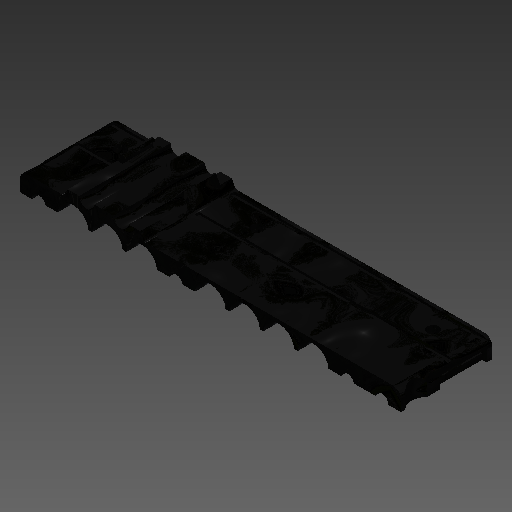
# Autodesk Inventor part: 3d_LM - Pinza 2
Saved by Autodesk Inventor 2018.3 (Build 223284000, 284)
## iProperties
Created: 2026-02-09
Part Number: 3d_LM - Pinza 2
Material: PA12 SLS 3D Print
Document SubType Name: Modeling
Designer: aca6
Density: 0.95 g/cm^3
Appearance: Black
Manufacturer-1: {"Name": "BERNARDO HENAREJOS ORENES (TECNOBRO)", "PartNumber": "3d_LM - Pinza 2", "Link": ""}
Manufacturer-2: {"Name": "MATERIALISE NV", "PartNumber": "3d_LM - Pinza 2", "Link": ""}
Manufacturer-3: {"Name": "", "PartNumber": "", "Link": ""}
Manufacturer-4: {"Name": "", "PartNumber": "", "Link": ""}
Manufacturer-5: {"Name": "", "PartNumber": "", "Link": ""}
Provider-1: {"Name": "", "PartNumber": "", "Link": ""}
Provider-2: {"Name": "", "PartNumber": "", "Link": ""}
Provider-3: {"Name": "", "PartNumber": "", "Link": ""}
Provider-4: {"Name": "", "PartNumber": "", "Link": ""}
Provider-5: {"Name": "", "PartNumber": "", "Link": ""}
Author: aca6
Comments: DIN-ISO-2768-mK
Autodesk Inventor part; units mm, degrees
ref_plane "YZ Plane" through (0, 0, 0) normal (1, 0, 0) x (0, 1, 0)
ref_plane "XZ Plane" through (0, 0, 0) normal (0, 1, 0) x (-1, 0, 0)
ref_plane "XY Plane" through (0, 0, 0) normal (0, 0, 1) x (1, 0, 0)
sketch "Sketch1" plane through (0, 0, 0) normal (0, 0, 1) x (1, 0, 0)
  arc A0 (-21.6, 0) -> (-23.4, 0) centre (-22.5, 0) ccw
  arc A1 (-15.975, 0) -> (-20.025, 0) centre (-18, 0) ccw
  arc A2 (-11.475, 0) -> (-15.525, 0) centre (-13.5, 0) ccw
  arc A3 (-6.975, 0) -> (-11.025, 0) centre (-9, 0) ccw
  arc A4 (-3.6, 0) -> (-5.4, 0) centre (-4.5, 0) ccw
  arc A5 (2.025, 0) -> (-2.025, 0) centre (0, 0) ccw
  arc A6 (6.525, 0) -> (2.475, 0) centre (4.5, 0) ccw
  arc A7 (11.025, 0) -> (6.975, 0) centre (9, 0) ccw
  arc A8 (15.525, 0) -> (11.475, 0) centre (13.5, 0) ccw
  arc A9 (18.875, 0) -> (17.125, 0) centre (18, 0) ccw
  arc A10 (23.375, 0) -> (21.625, 0) centre (22.5, 0) ccw
  line L0 (-25, 0) -> (-25, 1.5)
  line L1 (-25, 0) -> (25, 0)
  line L2 (25, 0) -> (25, 1.5)
  arc A11 (25, 1.5) -> (24, 2.5) centre (24, 1.5) ccw
  arc A12 (-24, 2.5) -> (-25, 1.5) centre (-24, 1.5) ccw
  line L3 (-8.467, 2.5) -> (24, 2.5)
  line L4 (-19.1661, 2.65) -> (-18.6985, 3.46)
  line L5 (-18.6985, 3.46) -> (-9.1945, 3.46)
  line L6 (-9.1945, 3.46) -> (-8.7268, 2.65)
  line L7 (-9.1945, 3.46) -> (-8.2592, 3.46) construction
  arc A13 (-8.7268, 2.65) -> (-8.467, 2.5) centre (-8.467, 2.8) ccw
  line L8 (-19.4259, 2.5) -> (-24, 2.5)
  arc A14 (-19.4259, 2.5) -> (-19.1661, 2.65) centre (-19.4259, 2.8) ccw
  line L9 (0, 0) -> (0, 12.7088) construction
  point P0 (-19.2527, 2.5)
  point P1 (-8.6402, 2.5)
  dimension "d1" = 1.8
  dimension "d2" = 4.5
  dimension "d3" = 4.5
  dimension "d4" = 4.5
  dimension "d5" = 4.5
  dimension "d6" = 4.5
  dimension "d7" = 4.5
  dimension "d8" = 4.5
  dimension "d9" = 4.5
  dimension "d10" = 4.5
  dimension "d11" = 4.5
  dimension "d12" = 4.05
  dimension "d13" = 4.05
  dimension "d14" = 4.05
  dimension "d15" = 1.8
  dimension "d16" = 4.05
  dimension "d17" = 4.05
  dimension "d18" = 4.05
  dimension "d19" = 4.05
  dimension "d20" = 1.75
  dimension "d21" = 1.75
  dimension "d22" = 2.5
  dimension "d23" = 50
  dimension "d24" = 1.5
  dimension "d25" = 1.5
  dimension "d26" = 1
  dimension "d27" = 1
  dimension "d29" = 120
  dimension "d32" = 9.504
  dimension "d33" = 60
  dimension "d67" = 0.96
  dimension "d68" = 0.3
  dimension "d69" = 0.3
  dimension "d70" = 33.467
  dimension "d71" = 5.5741
  constraints: 30 point on circle, 18 end point, 15 centre point, 9 tangent, 6 point on line, 4 vertical, 2 horizontal, 1 equal length, 39 other
  measures "d1" diameter of A0
  measures "d2" distance of A1.centre A0.centre
  measures "d3" distance of A2.centre A1.centre
  measures "d4" distance of A2.centre A3.centre
  measures "d5" distance of A3.centre A4.centre
  measures "d6" distance of A4.centre A5.centre
  measures "d7" distance of A5.centre A6.centre
  measures "d8" distance of A7.centre A6.centre
  measures "d9" distance of A8.centre A7.centre
  measures "d10" distance of A9.centre A8.centre
  measures "d11" distance of A10.centre A9.centre
  measures "d12" diameter of A1
  measures "d13" diameter of A2
  measures "d14" diameter of A3
  measures "d15" diameter of A4
  measures "d16" diameter of A5
  measures "d17" diameter of A6
  measures "d18" diameter of A7
  measures "d19" diameter of A8
  measures "d20" diameter of A9
  measures "d21" diameter of A10
  measures "d22" distance from line of A0.centre L0
  measures "d23" distance of L0.start L2.start
  measures "d24" distance of L0.start L0.end
  measures "d25" distance of L2.start L2.end
  measures "d26" radius of A11
  measures "d27" radius of A12
  measures "d29" angle of L3 L4
  measures "d32" distance of L4.end L5.end
  measures "d33" angle of L6 L7
  measures "d67" distance from line of L3 L5.end
  measures "d68" radius of A13
  measures "d69" radius of A14
  measures "d70" distance from line of L2 L3.start
  measures "d71" distance from line of L0 L8.start
extrude "Extrusion1" add sketch "Sketch1" along normal blind 12 contours A0 L1 L0 A12 L8 A14 L4 L5 L6 A13 L3 A11 L2 A10 A9 A8 A7 A6 A5 A4 A3 A2 A1
sketch "Sketch2" plane through (0, 0, 12) normal (0, 0, 1) x (1, 0, 0)
  line L0 (-9.1945, 3.46) -> (-18.6985, 3.46) projected
  point P0 (0, 0)
  point P1 (-16.1965, 3.46)
  point P2 (-11.6965, 3.46)
  dimension "d39" = 4.5
  dimension "d40" = 2.502
  constraints: 2 point on line
  measures "d39" distance of point (-11.696, 3.46) point (-16.196, 3.46)
  measures "d40" distance of L0.end point (-16.196, 3.46)
hole "Hole1" at (-16.1965, 3.46, 12) at (-11.6965, 3.46, 12) direction (0, 0, -1) diameter 2 end through all
sketch "Sketch3" plane through (24, 2.5, 12) normal (0, 1, 0) x (1, 0, 0)
  line L0 (0.714, 6.4) -> (-32.467, 6.4)
  line L1 (-32.467, 6.4) -> (-32.467, 7)
  line L2 (-32.467, 7) -> (0.714, 7)
  line L3 (0.714, 7) -> (0.714, 6.4)
  line L4 (-32.467, 11) -> (0.714, 11)
  line L5 (0.714, 11) -> (0.714, 11.6)
  line L6 (0.714, 11.6) -> (-32.467, 11.6)
  line L7 (-32.467, 11.6) -> (-32.467, 11)
  line L8 (1, 12) -> (1, 0) projected
  line L9 (0, 12) -> (-32.467, 12) projected
  line L10 (-43.4259, 6.4) -> (-48.29, 6.4)
  line L11 (-48.29, 6.4) -> (-48.29, 7)
  line L12 (-48.29, 7) -> (-43.4259, 7)
  line L13 (-43.4259, 7) -> (-43.4259, 6.4)
  line L14 (-43.4259, 11.6) -> (-48.29, 11.6)
  line L15 (-48.29, 11.6) -> (-48.29, 11)
  line L16 (-48.29, 11) -> (-43.4259, 11)
  line L17 (-43.4259, 11) -> (-43.4259, 11.6)
  line L18 (-49, 12) -> (-49, 0) projected
  point P0 (-24, 12)
  point P1 (-32.5535, 12.5)
  point P2 (-32.467, 12)
  point P3 (-43.4259, 12)
  dimension "d48" = 0.286
  dimension "d49" = 0.286
  dimension "d50" = 0.6
  dimension "d51" = 0.6
  dimension "d57" = 0.4
  dimension "d58" = 4
  dimension "d79" = 0.71
  constraints: 32 end point, 8 parallel, 5 point on line, 4 horizontal, 4 horizontal alignment, 4 perpendicular, 1 other
  measures "d48" distance between parallel lines of L8 L3
  measures "d49" distance between parallel lines of L8 L5
  measures "d50" distance of L2.end L0.start
  measures "d51" distance of L4.end L5.end
  measures "d58" distance between parallel lines of L2 L4
  measures "d79" distance between parallel lines of L18 L11
extrude "Extrusion2" cut sketch "Sketch3" against normal blind 0.3
ref_plane "Work Plane1" through (-2.9282, 3.7996, 12.5) normal (0, 1, 0) x (1, 0, 0)
sketch "Sketch4" plane through (-2.9282, 2.5, 12.5) normal (0, 1, 0) x (1, 0, 0)
  line L0 (27.9282, 12.5495) -> (27.9282, 3.2148)
  line L1 (26.9282, 11.5) -> (-5.5388, 11.5) projected
  line L2 (27.9282, 12.5) -> (27.9282, 0.5) projected
  line L3 (-22.0718, 12.5) -> (-22.0718, 0.5) projected
  point P0 (2.9282, 12.5)
  point P1 (-17.8838, 9.5)
  point P2 (0.1157, 9.5)
  point P3 (23.1782, 9.5)
  dimension "d54" = 4.75
  dimension "d72" = 2
  dimension "d121" = 4.188
  dimension "d122" = 23.0625
  constraints: 2 end point, 2 horizontal alignment, 2 point on line
  measures "d54" distance from line of L0 point (23.178, 9.5)
  measures "d72" distance from line of L1 point (23.178, 9.5)
  measures "d121" distance from line of L3 point (-17.884, 9.5)
  measures "d122" distance of point (0.116, 9.5) point (23.178, 9.5)
hole "Hole2" at (-20.812, 2.5, 3) at (-2.8125, 2.5, 3) at (20.25, 2.5, 3) direction (0, -1, 0) diameter 1.5 end through all both
sketch "Sketch5" plane through (-8.467, 2.5, 12) normal (0, 1, 0) x (1, 0, 0)
  circle A0 centre (34.867, 2.0003) radius 2
  line L0 (32.467, 0) -> (33.467, 0) projected
  line L1 (33.467, 12) -> (33.467, 0) projected
  line L2 (33.467, 0) -> (33.467, 0.572)
  point P0 (8.467, 12)
  dimension "d73" = 4
  dimension "d75" = 1.4
  dimension "d76" = 0.572
  constraints: 2 end point, 1 point on line, 3 other
  measures "d75" distance from line of L1 point (34.867, 2)
  measures "d76" distance of L0.end L2.end
extrude "Extrusion3" cut sketch "Sketch5" against normal blind 7.05
mirror "Mirror1" about plane through (0, 0, 0) normal (1, 0, 0) of "Extrusion3"
ref_plane "Work Plane2" through (0, 0, 1.5) normal (0, 0, -1) x (-1, 0, 0)
sketch "Sketch6" plane through (0, 0, 1.5) normal (0, 0, -1) x (-1, 0, 0)
  line L0 (8.7268, 2.65) -> (9.1945, 3.46) projected
  line L1 (9.1945, 3.46) -> (9.7718, 4.46)
  line L2 (9.1945, 3.46) -> (10.6965, 3.46) projected
  line L3 (9.7718, 4.46) -> (9.9768, 4.46)
  line L4 (9.9768, 4.46) -> (10.1968, 4.16)
  line L5 (10.1968, 4.16) -> (9.8968, 4.16)
  line L6 (9.8968, 4.16) -> (9.8968, 3.46)
  line L7 (9.1945, 3.46) -> (10.6965, 3.46) projected
  line L8 (9.8968, 3.46) -> (9.1945, 3.46)
  line L9 (12.6965, 3.46) -> (15.1965, 3.46) projected
  line L10 (13.9465, 3.46) -> (13.9465, 5.3261) construction
  line L11 (17.1965, 3.46) -> (18.6985, 3.46) projected
  line L12 (18.6985, 3.46) -> (18.1211, 4.46)
  line L13 (18.6985, 3.46) -> (19.8532, 3.46) construction
  line L14 (18.1211, 4.46) -> (17.9161, 4.46)
  line L15 (17.9161, 4.46) -> (17.6961, 4.16)
  line L16 (17.6961, 4.16) -> (17.9961, 4.16)
  line L17 (17.9961, 4.16) -> (17.9961, 3.46)
  line L18 (17.9961, 3.46) -> (18.6985, 3.46)
  point P0 (0, 0)
  dimension "d81" = 1
  dimension "d82" = 0.205
  dimension "d83" = 126.25
  dimension "d84" = 0.3
  dimension "d85" = 0.3
  dimension "d94" = 120
  dimension "d95" = 1
  dimension "d96" = 0.205
  dimension "d97" = 53.75
  dimension "d98" = 53.75
  dimension "d99" = 0.3
  dimension "d100" = 0.3
  constraints: 28 end point, 5 horizontal, 3 collinear, 2 perpendicular, 2 point on line, 2 vertical, 1 equal length, 1 midpoint, 1 other
  measures "d81" distance from line of L2 L1.end
  measures "d82" distance of L1.end L3.end
  measures "d83" angle of L3 L4
  measures "d84" distance from line of L3 L4.end
  measures "d85" distance of L4.end L5.end
  measures "d94" angle of L13 L12
  measures "d95" distance from line of L11 L12.end
  measures "d96" distance of L12.end L14.end
  measures "d97" angle of L5 L4
  measures "d98" angle of L15 L16
  measures "d99" distance from line of L14 L15.end
  measures "d100" distance of L15.end L16.end
extrude "Extrusion4" add sketch "Sketch6" against normal blind 4
ref_plane "Work Plane4" through (0, 0, 0.45) normal (0, 0, -1) x (-1, 0, 0)
sketch "Sketch7" plane through (0, 0, 0.45) normal (0, 0, -1) x (-1, 0, 0)
  line L0 (24.9987, 1.55) -> (24.4667, 1.55)
  line L1 (25, 0) -> (20.025, 0) projected
  arc A0 (15.1965, 3.46) -> (17.1965, 3.46) centre (16.1965, 3.46) ccw projected
  line L2 (12.6965, 3.46) -> (15.1965, 3.46) projected
  arc A1 (10.6965, 3.46) -> (12.6965, 3.46) centre (11.6965, 3.46) ccw projected
  line L3 (9.1945, 3.46) -> (10.6965, 3.46) projected
  line L4 (8.7268, 2.65) -> (9.1945, 3.46) projected
  arc A2 (8.467, 2.5) -> (8.7268, 2.65) centre (8.467, 2.8) ccw projected
  line L5 (-24, 2.5) -> (8.467, 2.5) projected
  arc A3 (-24, 2.5) -> (-25, 1.5) centre (-24, 1.5) ccw projected
  line L6 (-25, 0) -> (-25, 1.5) projected
  line L7 (-23.375, 0) -> (-25, 0) projected
  arc A4 (-21.625, 0) -> (-23.375, 0) centre (-22.5, 0) ccw projected
  line L8 (-18.875, 0) -> (-21.625, 0) projected
  arc A5 (-17.125, 0) -> (-18.875, 0) centre (-18, 0) ccw projected
  line L9 (-15.525, 0) -> (-17.125, 0) projected
  arc A6 (-11.475, 0) -> (-15.525, 0) centre (-13.5, 0) ccw projected
  line L10 (-11.025, 0) -> (-11.475, 0) projected
  arc A7 (-6.975, 0) -> (-11.025, 0) centre (-9, 0) ccw projected
  line L11 (-6.525, 0) -> (-6.975, 0) projected
  arc A8 (-2.475, 0) -> (-6.525, 0) centre (-4.5, 0) ccw projected
  line L12 (-2.025, 0) -> (-2.475, 0) projected
  arc A9 (2.025, 0) -> (-2.025, 0) centre (0, 0) ccw projected
  line L13 (3.6, 0) -> (2.025, 0) projected
  arc A10 (5.4, 0) -> (3.6, 0) centre (4.5, 0) ccw projected
  line L14 (6.975, 0) -> (5.4, 0) projected
  arc A11 (11.025, 0) -> (6.975, 0) centre (9, 0) ccw projected
  line L15 (11.475, 0) -> (11.025, 0) projected
  arc A12 (15.525, 0) -> (11.475, 0) centre (13.5, 0) ccw projected
  line L16 (15.975, 0) -> (15.525, 0) projected
  arc A13 (20.025, 0) -> (15.975, 0) centre (18, 0) ccw projected
  line L17 (25, 0) -> (23.4, 0) projected
  line L18 (25, 1.5) -> (25, 0) projected
  arc A14 (25, 1.5) -> (24, 2.5) centre (24, 1.5) ccw projected
  line L19 (19.4259, 2.5) -> (24, 2.5) projected
  arc A15 (19.1661, 2.65) -> (19.4259, 2.5) centre (19.4259, 2.8) ccw projected
  line L20 (18.6985, 3.46) -> (19.1661, 2.65) projected
  line L21 (17.1965, 3.46) -> (18.6985, 3.46) projected
  line L22 (24.4667, 1.55) -> (24.124, 0.7504)
  line L23 (24.4667, 1.55) -> (25.3367, 1.55) construction
  line L24 (24.124, 0.7504) -> (24.4, 0.7504)
  line L25 (24.4, 0.7504) -> (24.4, 0)
  line L26 (24.4, 0) -> (25, 0)
  arc A16 (25, 1.5) -> (24, 2.5) centre (24, 1.5) ccw projected
  line L27 (25, 0) -> (25, 1.5)
  line L28 (21.6, 0) -> (20.025, 0) projected
  arc A17 (23.4, 0) -> (21.6, 0) centre (22.5, 0) ccw projected
  point P0 (0, 0)
  dimension "d102" = 1.55
  dimension "d103" = 0.532
  dimension "d104" = 113.2
  dimension "d105" = 0.87
  dimension "d106" = 0.276
  constraints: 14 end point, 3 horizontal, 2 perpendicular, 2 tangent, 1 collinear, 1 equal length, 1 point on circle, 1 point on line
  measures "d102" distance between parallel lines of L1 L0
  measures "d103" distance of L0.start L0.end
  measures "d104" angle of L22 L23
  measures "d105" distance of L0.end L22.end
  measures "d106" distance of L22.end L24.end
extrude "Extrusion5" cut sketch "Sketch7" against normal blind 6.1 contours A14 L18 L1 L25 L24 L22 L0
sketch "Sketch8" plane through (0, 0, 12) normal (0, 0, 1) x (1, 0, 0)
  line L0 (-22, 0) -> (23, 0)
  line L1 (23, 0) -> (23, 0.175)
  line L2 (23, 0.175) -> (-22, 0.175)
  line L3 (-22, 0.175) -> (-22, 0)
  line L4 (25, 0) -> (25, 1.5) projected
  point P0 (0, 0)
  point P1 (21.625, 0)
  dimension "d109" = 0.175
  dimension "d110" = 45
  dimension "d111" = 2
  constraints: 8 end point, 2 parallel, 1 horizontal, 1 perpendicular, 1 point on line
  measures "d109" distance of L1.end L0.end
  measures "d110" distance of L0.start L0.end
  measures "d111" distance between parallel lines of L4 L1
extrude "Extrusion6" cut sketch "Sketch8" against normal through all
ref_plane "Work Plane5" through (0, 0, 0.75) normal (0, 0, -1) x (-1, 0, 0)
sketch "Sketch9" plane through (0, 0, 0.75) normal (0, 0, -1) x (-1, 0, 0)
  line L0 (24.9987, 1.55) -> (24.4667, 1.55)
  line L1 (25, 0) -> (24.25, 0)
  line L2 (25, 1.5) -> (25, 0)
  line L3 (24.4667, 1.55) -> (24.124, 0.7504)
  line L4 (24.4667, 1.55) -> (25.3367, 1.55) construction
  line L5 (24.124, 0.7504) -> (24.4, 0.7504)
  line L6 (24.4, 0.7504) -> (24.4, 0)
  line L7 (24.4, 0) -> (25, 0)
  line L8 (25, 0) -> (25, 1.5)
  line L9 (0, 0) -> (0, 5.6827) construction
  line L10 (-24.9987, 1.55) -> (-24.4667, 1.55)
  line L11 (-24.4, 0.7504) -> (-24.4, 0)
  line L12 (-25, 0.7504) -> (-25, 0)
  line L13 (-24.4, 0) -> (-25, 0)
  line L14 (-25, 0) -> (-25, 1.5)
  line L15 (-24.4667, 1.55) -> (-25.3367, 1.55) construction
  line L16 (-25, 0) -> (-24.25, 0)
  line L17 (-24.124, 0.7504) -> (-24.4, 0.7504)
  line L18 (-24.4667, 1.55) -> (-24.124, 0.7504)
  arc A0 (-24, 2.5) -> (-25, 1.5) centre (-24, 1.5) ccw projected
  arc A1 (-24.9987, 1.55) -> (-25, 1.5) centre (-24, 1.5) ccw
  point P0 (24.25, 0)
  point P1 (24, 1.5)
  point P2 (24, 1.5)
  point P3 (-24.25, 0)
  point P4 (-24, 1.5)
  point P5 (-24, 1.5)
  dimension "d115" = 0.532
  dimension "d116" = 113.2
  dimension "d117" = 0.87
  dimension "d118" = 0.276
  constraints: 38 end point, 12 symmetric about line, 4 point on line, 3 horizontal, 3 vertical, 2 point on circle, 1 centre point, 1 coincident, 1 collinear, 1 equal length, 1 perpendicular, 1 other
  measures "d115" distance of L0.start L0.end
  measures "d116" angle of L3 L4
  measures "d117" distance of L0.end L5.start
  measures "d118" distance of L5.start L6.start
extrude "Extrusion7" cut sketch "Sketch9" against normal blind 6.1
body "Solid1"
